Autodesk Inventor part; units mm, degrees
(part 2 of 2)
sketch "Esquisse13" plane through (32, -1, -9.8) normal (1, 0, 0) x (0, 0, -1)
  line L0 (0.2, -23.9) -> (0.2, -43.9)
  line L1 (0.2, -43.9) -> (-24.8, -43.9)
  line L2 (-9.8, -3.1) -> (-9.8, -9.1) projected
  line L3 (-9.8, -9.1) -> (-9.8, -3.1) projected
  line L4 (-9.8, -25.9) -> (-9.8, -31.9) projected
  line L5 (-9.8, -31.9) -> (-9.8, -25.9) projected
  line L6 (-9.8, -25.9) -> (-9.8, -31.9) projected
  line L7 (-9.8, -31.9) -> (-9.8, -25.9) projected
  line L8 (-9.8, 16.9) -> (-9.8, 22.9) projected
  line L9 (-9.8, 22.9) -> (-9.8, 16.9) projected
  line L10 (-9.8, 45.7) -> (-9.8, 39.7) projected
  line L11 (-9.8, 39.7) -> (-9.8, 45.7) projected
  line L12 (-9.8, 45.7) -> (-9.8, 39.7) projected
  line L13 (-9.8, 39.7) -> (-9.8, 45.7) projected
  line L14 (-9.8, -0.5) -> (-9.8, -3.5) projected
  line L15 (-9.8, -0.5) -> (-9.8, -3.5) projected
  line L16 (-9.8, 17.3) -> (-9.8, 14.3) projected
  line L17 (-9.8, 17.3) -> (-9.8, 14.3) projected
  line L18 (-9.8, -9.1) -> (-9.8, -33.9) projected
  line L19 (-9.8, -33.9) -> (-9.8, -9.1) projected
  line L20 (-9.8, 1) -> (-9.8, -9.1) projected
  line L21 (-9.8, 12.8) -> (-9.8, 1) projected
  line L22 (-9.8, 22.9) -> (-9.8, 12.8) projected
  line L23 (-9.8, 22.9) -> (-9.8, 47.7) projected
  line L24 (-9.8, 47.7) -> (-9.8, 22.9) projected
  line L25 (-9.8, 12.8) -> (-9.8, 22.9) projected
  line L26 (-9.8, 1) -> (-9.8, 12.8) projected
  line L27 (-9.8, -9.1) -> (-9.8, 1) projected
  line L28 (0.2, -23.9) -> (-9.8, -23.9)
  line L29 (-9.8, -23.9) -> (-9.8, -33.9)
  line L30 (-9.8, -33.9) -> (-15.8, -33.9)
  line L31 (-15.8, -33.9) -> (-15.8, -27.2333)
  line L32 (-15.8, -27.2333) -> (-24.8, -33.9)
  line L33 (-24.8, -33.9) -> (-24.8, -46.4321) construction
  arc A0 (-24.8, -33.9) -> (-24.8, -43.9) centre (-24.8, -38.9) ccw
  line L34 (-9.8, -25.9) -> (-9.8, -26.1) projected
  line L35 (-9.8, -26.1) -> (-9.8, -25.9) projected
  line L36 (-9.8, -31.9) -> (-9.8, -31.7) projected
  line L37 (-9.8, -31.7) -> (-9.8, -31.9) projected
  line L38 (-9.8, -31.9) -> (-9.8, -31.7) projected
  line L39 (-9.8, -31.7) -> (-9.8, -31.9) projected
  line L40 (-9.8, -25.9) -> (-9.8, -26.1) projected
  line L41 (-9.8, -26.1) -> (-9.8, -25.9) projected
  line L42 (-9.8, -31.9) -> (-9.8, -31.7) projected
  line L43 (-9.8, -31.7) -> (-9.8, -31.9) projected
  line L44 (-9.8, -31.9) -> (-9.8, -31.7) projected
  line L45 (-9.8, -31.7) -> (-9.8, -31.9) projected
  line L46 (-9.8, 39.7) -> (-9.8, 39.9) projected
  line L47 (-9.8, 39.9) -> (-9.8, 39.7) projected
  line L48 (-9.8, 39.7) -> (-9.8, 39.9) projected
  line L49 (-9.8, 39.9) -> (-9.8, 39.7) projected
  line L50 (-9.8, 45.7) -> (-9.8, 45.5) projected
  line L51 (-9.8, 45.5) -> (-9.8, 45.7) projected
  line L52 (-9.8, 39.7) -> (-9.8, 39.9) projected
  line L53 (-9.8, 39.9) -> (-9.8, 39.7) projected
  line L54 (-9.8, 39.7) -> (-9.8, 39.9) projected
  line L55 (-9.8, 39.9) -> (-9.8, 39.7) projected
  line L56 (-9.8, 45.7) -> (-9.8, 45.5) projected
  line L57 (-9.8, 45.5) -> (-9.8, 45.7) projected
  point P0 (0.2, -25.9)
  dimension "d70" = 6
  dimension "d71" = 25
  dimension "d74" = 10
  dimension "d75" = 6.6667
  dimension "d76" = 0
  dimension "d82" = 20
  constraints: 16 end point, 5 perpendicular, 2 parallel, 2 point on circle, 2 point on line, 1 centre point, 1 coincident, 1 collinear, 1 tangent
  measures "d70" distance of L29.end L30.end
  measures "d71" distance of L0.end L1.end
  measures "d74" distance of L18.end L28.end
  measures "d75" distance of L30.end L31.end
  measures "d76" vertical distance of L32.end L30.end
  measures "d82" distance of L0.start L0.end
extrude "Extrusion11" add sketch "Esquisse13" along normal mid plane 6 separate body
mirror "Symétrie5" about plane through (-10.8, 5.9, -9.8) normal (0, 1, 0) of "Extrusion11" bodies 7
sketch "Esquisse14" plane through (-2.8, 44.7, -81.6) normal (0, 1, 0) x (1, 0, 0)
  circle A0 centre (10, -10) radius 3
  line L0 (0, 0) -> (69.6, 0) projected
  line L1 (0, -12.82) -> (0, 0) projected
  point P0 (2.8, -81.6)
  dimension "d254" = 6
  dimension "d255" = 10
  dimension "d256" = 10
  constraints: 1 centre point
  measures "d254" diameter of A0
  measures "d255" distance from line of L0 A0.centre
  measures "d256" distance from line of L1 A0.centre
extrude "Extrusion12" cut sketch "Esquisse14" against normal blind 6 bodies 4
sketch "Esquisse15" plane through (28.5, -32.9, 6) normal (0, -1, 0) x (1, 0, 0)
  line L0 (-6.5, -37) -> (-6.5, -31)
  line L1 (13.5, -31) -> (13.5, -37)
  line L2 (13.5, -37) -> (3.5, -37) construction
  line L3 (3.5, -37) -> (-6.5, -37) construction
  line L4 (3.5, 17.52) -> (3.5, -105.12) construction
  line L5 (12.8, -37) -> (12.8, -36.8)
  line L6 (12.8, -36.8) -> (11.8, -36.8)
  line L7 (11.8, -36.8) -> (11.8, -37)
  line L8 (-4.8, -37) -> (-4.8, -36.8)
  line L9 (-4.8, -36.8) -> (-5.8, -36.8)
  line L10 (-5.8, -36.8) -> (-5.8, -37)
  line L11 (4, -31) -> (4, -31.2)
  line L12 (4, -31.2) -> (3, -31.2)
  line L13 (3, -31.2) -> (3, -31)
  line L14 (13.5, -37) -> (12.8, -37)
  line L15 (11.8, -37) -> (-4.8, -37)
  line L16 (-5.8, -37) -> (-6.5, -37)
  line L17 (-6.5, -31) -> (3, -31)
  line L18 (4, -31) -> (13.5, -31)
  line L19 (13.5, -37) -> (3.5, -37) construction
  line L20 (3.5, -37) -> (-6.5, -37) construction
  point P0 (-28.5, -6)
  point P1 (6.5, -16)
  dimension "d259" = 20
  dimension "d260" = 6
  dimension "d261" = 15
  dimension "d262" = 0.2
  dimension "d263" = 0.2
  dimension "d264" = 1
  dimension "d265" = 1
  dimension "d266" = 1
  dimension "d267" = 0.7
  dimension "d268" = 0.7
  dimension "d269" = 9.5
  constraints: 40 end point, 15 perpendicular, 7 collinear, 7 parallel, 7 point on line, 3 horizontal, 1 midpoint, 1 vertical
  measures "d259" distance of L1.end L0.start
  measures "d260" distance of L0.start L0.end
  measures "d261" vertical distance of point (6.5, -16) L1.start
  measures "d262" distance of L6.end L7.end
  measures "d263" distance of L12.end L13.end
  measures "d264" distance of L5.end L6.end
  measures "d265" distance of L8.end L9.end
  measures "d266" distance of L11.end L12.end
  measures "d267" horizontal distance of L5.end L1.end
  measures "d268" horizontal distance of L0.start L9.end
  measures "d269" horizontal distance of L1.start L11.end
extrude "Extrusion13" cut sketch "Esquisse15" against normal blind 6 bodies 4
equation "\"d0\" = epaisseur"
equation "\"d1\" = 0.5 * L_fente"
equation "\"d2\" = epaisseur"
equation "\"d3\" = 0.5 * largeur"
equation "\"d4\" = dvis"
equation "\"d5\" = dvis"
equation "\"d6\" = dvis"
equation "\"d7\" = epaisseur"
equation "\"d11\" = epaisseur"
equation "\"d28\" = epaisseur"
equation "\"d29\" = epaisseur"
equation "\"d33\" = epaisseur + marge_attache_carte"
equation "\"d35\" = 0.5 * L_attache_carte"
equation "\"d30\" = epaisseur"
equation "\"d36\" = epaisseur"
equation "\"d37\" = epaisseur"
equation "\"d38\" = 0.5 * L_cubi"
equation "\"d39\" = 0.25 * largeur_cubi - 0.5 * taille_trou"
equation "\"d40\" = 0.25 * largeur_cubi - 0.5 * taille_trou"
equation "\"d41\" = taille_trou"
equation "\"d43\" = taille_trou"
equation "\"epaisseur\" = 6"
equation "\"ecartement\" = 25"
equation "\"dvis\" = 3"
equation "\"largeur\" = 32"
equation "\"L_attache_carte\" = 15"
equation "\"marge_attache_carte\" = 5"
equation "\"taille_trou\" = 7"
equation "\"L_moteur\" = 28.3"
equation "\"largeur_cubi\" = 81.6"
equation "\"marge_trou\" = 2"
equation "\"L_cubi\" = 81.6"
equation "\"H_cubi\" = 81.6"
equation "\"epaisseur_wheel\" = 9"
equation "\"H_nez\" = 25"
equation "\"chanfrein\" = 0.5"
equation "\"H_trou_int\" = 0.2"
equation "\"L_trou_int\" = 1"
equation "\"pos_trou_int_1\" = 0.7"
equation "\"pos_trou_int_2\" = 3"
equation "\"epaisseur_metabois\" = 3"
equation "\"L_metabois\" = 8.2"
equation "\"epaisseur_modules\" = 6"
equation "\"L_fente\" = 30"
